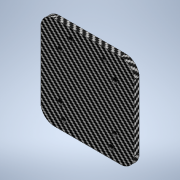
# Autodesk Inventor part: retractable_landing_skids_adapter_plate
Saved by Autodesk Inventor 2020.2 (Build 242310000, 310)
## iProperties
Created: 2020-10-27
Part Number: retractable_landing_skids_adapter_plate
Material: CFRP
Document SubType Name: Modeling
Designer: Krishna Makhija
Density: 1.43 g/cm^3
Appearance: Carbon Fiber
Author: Krishna Makhija
Autodesk Inventor part; units mm, degrees
ref_plane "YZ Plane" through (0, 0, 0) normal (1, 0, 0) x (0, 1, 0)
ref_plane "XZ Plane" through (0, 0, 0) normal (0, 1, 0) x (-1, 0, 0)
ref_plane "XY Plane" through (0, 0, 0) normal (0, 0, 1) x (1, 0, 0)
sketch "Sketch1" plane through (0, 0, 0) normal (0, 0, 1) x (1, 0, 0)
  point P0 (0, 0)
sketch "Sketch2" plane through (0, 0, 0) normal (0, 0, 1) x (1, 0, 0)
  line L0 (27.5, -27.5002) -> (-27.5, -27.5002)
  line L1 (-27.5, -27.5002) -> (-27.5, 27.5002)
  line L2 (-27.5, 27.5002) -> (27.5, 27.5002)
  line L3 (27.5, 27.5002) -> (27.5, -27.5002)
  circle A0 centre (16, 13.5) radius 1.5
  circle A1 centre (-16, 13.5) radius 1.5
  circle A2 centre (-16, -13.5) radius 1.5
  circle A3 centre (16, -13.5) radius 1.5
  circle A4 centre (14, -21.5) radius 1.5
  circle A5 centre (-14, -21.5) radius 1.5
  circle A6 centre (10, 21.5) radius 1.2498
  circle A7 centre (-10, 21.5) radius 1.2498
  constraints: 8 centre point, 8 end point, 2 parallel, 1 horizontal, 1 perpendicular
extrude "Extrusion3" add sketch "Sketch2" along normal blind 3
fillet "Fillet3" radius 8 4 edges at (27.5, 27.5002, 1.5) (-27.5, 27.5002, 1.5) (27.5, -27.5002, 1.5) (-27.5, -27.5002, 1.5)
body "Solid3"
